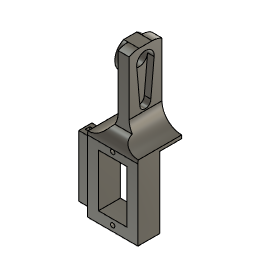
Final Assembly (Autodesk Fusion 360 archive; units mm, degrees)
design "hip_right_v2"
Autodesk Fusion 360 part; units mm, degrees
(part 1 of 2)
sketch "Sketch1" plane through (0, 0, 0) normal (1, 0, 0) x (0, 1, 0)
  line L0 (0, 0) -> (25, 0)
  line L1 (25, 0) -> (25, 35)
  line L2 (25, 35) -> (0, 35)
  line L3 (0, 35) -> (0, 0)
  dimension "d1" = 25
  dimension "d2" = 35
  constraint horizontal L0
  constraint vertical L1
  constraint horizontal L2
  constraint vertical L3
  constraint coincident L0.start L3.end
  measures "d1" distance of L0.start L0.end
  measures "d2" distance of L0.start L2.end
extrude "Extrude1" add sketch "Sketch1" along normal blind 5
sketch "Sketch2" plane through (5, 0, 0) normal (1, 0, 0) x (0, 1, 0)
  line L0 (0, 35) -> (0, 0)
  line L1 (0, 0) -> (25, 0)
  line L2 (25, 0) -> (25, 35)
  line L3 (25, 35) -> (0, 35)
  circle A0 centre (12.4718, 28.6693) radius 4
  line L4 (12.4317, 32.6691) -> (12.4317, 9.6691)
  circle A1 centre (12.4317, 12.1237) radius 2.5
  line L5 (14.9305, 12.1994) -> (16.454, 28.2923)
  line L6 (8.4897, 28.2923) -> (9.9414, 11.9031)
  line L7 (5, 35) -> (20, 35)
  line L8 (20, 35) -> (20, 0)
  line L9 (20, 0) -> (5, 0)
  line L10 (5, 0) -> (5, 35)
  dimension "d5" = 8
  dimension "d6" = 23
  dimension "d7" = 5
  constraint coincident A0 L4.start
  constraint vertical L4
  constraint coincident L4 A1.centre
  constraint coincident A1 L5.start
  constraint coincident A0 L5.end
  constraint tangent A0 L5
  constraint coincident A0 L6.start
  constraint coincident A1 L6.end
  constraint tangent A1 L6
  constraint horizontal L7
  constraint vertical L8
  constraint horizontal L9
  constraint vertical L10
  measures "d5" diameter of A0
  measures "d6" distance of L4.start L4.end
  measures "d7" diameter of A1
extrude "Extrude3" cut sketch "Sketch2" against normal blind 3 contours A0 L4 A1 L5 | A0 L4 A1 L6 | A1
extrude "Extrude2" cut sketch "Sketch2" against normal blind 5 contours A0 L4 | A0 L4
sketch "Sketch3" plane through (0, 0, 0) normal (-1, 0, 0) x (0, -1, 0)
  circle A0 centre (-12.4718, 28.6693) radius 4
  line L0 (0, 0) -> (0, 35)
  line L1 (0, 35) -> (-25, 35)
  line L2 (-25, 35) -> (-25, 0)
  line L3 (-25, 0) -> (0, 0)
  circle A1 centre (-12.4718, 28.6693) radius 4
  circle A2 centre (-12.4718, 28.6693) radius 7
  dimension "d12" = 14
  constraint concentric A0 A1
  constraint concentric A1 A2
  measures "d12" diameter of A2
extrude "Extrude4" add sketch "Sketch3" along normal blind 2 contours L1 A2 picked at (-12.3722, 34.2194)
sketch "Sketch4" plane through (0, 0, 0) normal (0, 0, -1) x (1, 0, 0)
  line L0 (0, 0) -> (0, -25)
  line L1 (0, -25) -> (5, -25)
  line L2 (5, -25) -> (5, 0)
  line L3 (5, 0) -> (0, 0)
  line L4 (0, 0) -> (5, 0)
  line L5 (5, 0) -> (5, -25)
  line L6 (5, -25) -> (0, -25)
  line L7 (0, -25) -> (0, 0)
  constraint horizontal L4
  constraint vertical L5
  constraint horizontal L6
  constraint vertical L7
  constraint coincident L1.end L2.start
  constraint coincident L0.start L3.end
extrude "Extrude5" add sketch "Sketch4" along normal blind 34
sketch "Sketch5" plane through (5, 0, 0) normal (1, 0, 0) x (0, 1, 0)
  arc A0 (16.454, 28.2923) -> (8.4897, 28.2923) centre (12.4718, 28.6693) ccw
  line L0 (16.454, 28.2923) -> (14.9305, 12.1994)
  arc A1 (9.9414, 11.9031) -> (14.9305, 12.1994) centre (12.4317, 12.1237) ccw
  line L1 (9.9414, 11.9031) -> (8.4897, 28.2923)
  line L2 (0, 35) -> (0, -34)
  line L3 (0, -34) -> (25, -34)
  line L4 (25, -34) -> (25, 35)
  line L5 (25, 35) -> (0, 35)
  line L6 (25, -34) -> (0, -34)
  line L7 (0, -34) -> (0, 0)
  line L8 (0, 0) -> (25, 0)
  line L9 (25, 0) -> (25, -34)
  constraint horizontal L6
  constraint vertical L7
  constraint horizontal L8
  constraint vertical L9
  constraint coincident L7.end L8.start
  constraint coincident L3.end L4.start
extrude "Extrude6" add sketch "Sketch5" along normal blind 12 contours L2 L3 L4 L6 L7 L8 L9
sketch "Sketch6" plane through (0, 0, 0) normal (-1, 0, 0) x (0, -1, 0)
  arc A0 (-15.4588, 35) -> (-9.4848, 35) centre (-12.4718, 28.6693) ccw
  line L0 (-15.4588, 35) -> (-25, 35)
  line L1 (-25, 35) -> (-25, -34)
  line L2 (-25, -34) -> (0, -34)
  line L3 (0, -34) -> (0, 35)
  line L4 (0, 35) -> (-9.4848, 35)
  line L5 (-25, -34) -> (0, -34)
  line L6 (0, -34) -> (0, 0)
  line L7 (0, 0) -> (-25, 0)
  line L8 (-25, 0) -> (-25, -34)
  constraint horizontal L5
  constraint vertical L6
  constraint horizontal L7
  constraint vertical L8
  constraint coincident L6.end L7.start
  constraint coincident L1.end L2.start
extrude "Extrude7" add sketch "Sketch6" along normal blind 12 contours L1 L2 L3 L5 L6 L7 L8
sketch "Sketch7" plane through (0, 25, 0) normal (0, 1, 0) x (-1, 0, 0)
  line L0 (0, 0) -> (0, 35)
  line L1 (0, 35) -> (-5, 35)
  line L2 (-5, 35) -> (-5, 0)
  line L3 (-5, 0) -> (-17, 0)
  line L4 (-17, 0) -> (-17, -34)
  line L5 (-17, -34) -> (12, -34)
  line L6 (12, -34) -> (12, 0)
  line L7 (12, 0) -> (0, 0)
  line L8 (-2.5, 0) -> (-2.5, -34)
  line L9 (-2.5, -34) -> (-2.5, -29)
  line L10 (-2.5, -29) -> (4, -29)
  line L11 (4, -29) -> (-9, -29)
  line L12 (-9, -29) -> (-9, -5)
  line L13 (-9, -5) -> (4, -5)
  line L14 (4, -5) -> (4, -29)
  dimension "d21" = 5
  dimension "d22" = 6.5
  dimension "d23" = 13
  dimension "d24" = 24
  constraint midpoint L5 L8.end
  constraint perpendicular L5 L9
  constraint perpendicular L9 L10
  constraint horizontal L11
  constraint vertical L12
  constraint horizontal L13
  constraint vertical L14
  measures "d21" distance of L8.end L9.end
  measures "d22" distance of L9.end L10.end
  measures "d23" distance of L10.end L11.end
  measures "d24" distance of L10.end L13.end
extrude "Extrude8" cut sketch "Sketch7" against normal blind 25 contours L8 L10 L11 L13 L14 | L8 L11 L12 L13
sketch "Sketch8" plane through (0, 25, 0) normal (0, 1, 0) x (-1, 0, 0)
  line L0 (-9, -29) -> (-9, -5)
  line L1 (-9, -5) -> (4, -5)
  line L2 (4, -5) -> (4, -29)
  line L3 (4, -29) -> (-9, -29)
  line L4 (0, 0) -> (0, 35)
  line L5 (0, 35) -> (-5, 35)
  line L6 (-5, 35) -> (-5, 0)
  line L7 (-5, 0) -> (-17, 0)
  line L8 (-17, 0) -> (-17, -34)
  line L9 (-17, -34) -> (12, -34)
  line L10 (12, -34) -> (12, 0)
  line L11 (12, 0) -> (0, 0)
  line L12 (-9, -5) -> (-14, -5)
  line L13 (-14, -5) -> (-14, 0)
  line L14 (-14, 0) -> (-9, 0)
  line L15 (-9, 0) -> (-9, -5)
  line L16 (4, -5) -> (9, -5)
  line L17 (9, -5) -> (9, 0)
  line L18 (9, 0) -> (4, 0)
  line L19 (4, 0) -> (4, -5)
  line L20 (9, 0) -> (12, 0)
  line L21 (12, 0) -> (12, -34)
  line L22 (12, -34) -> (9, -34)
  line L23 (9, -34) -> (9, 0)
  line L24 (-14, 0) -> (-17, 0)
  line L25 (-17, 0) -> (-17, -34)
  line L26 (-17, -34) -> (-14, -34)
  line L27 (-14, -34) -> (-14, 0)
  dimension "d27" = 5
  dimension "d28" = 5
  dimension "d29" = 5
  dimension "d30" = 5
  constraint horizontal L12
  constraint vertical L13
  constraint horizontal L14
  constraint vertical L15
  constraint coincident L0.end L1.start
  constraint horizontal L16
  constraint vertical L17
  constraint horizontal L18
  constraint vertical L19
  constraint coincident L1.end L2.start
  constraint horizontal L20
  constraint vertical L21
  constraint horizontal L22
  constraint vertical L23
  constraint coincident L9.end L10.start
  constraint horizontal L24
  constraint vertical L25
  constraint horizontal L26
  constraint vertical L27
  constraint coincident L8.end L9.start
  measures "d27" distance of L0.end L12.end
  measures "d28" distance of L0.end L14.end
  measures "d29" distance of L1.end L16.end
  measures "d30" distance of L1.end L18.end
extrude "Extrude9" cut sketch "Sketch8" against normal blind 25 contours L7 L8 L9 L13 L24 L25 L26 L27 | L9 L10 L11 L17 L20 L21 L22 L23
fillet "Fillet1" radius 9 2 edges at (5, 12.5, 0) (0, 12.5, 0)
sketch "Sketch9" plane through (0, 0, 0) normal (0, -1, 0) x (1, 0, 0)
  line L0 (9, -5) -> (9, -29)
  line L1 (9, -29) -> (-4, -29)
  line L2 (-4, -29) -> (-4, -5)
  line L3 (-4, -5) -> (9, -5)
  line L4 (-9, 0) -> (-9, -34)
  line L5 (-9, -34) -> (14, -34)
  line L6 (14, -34) -> (14, 0)
  arc A0 (5, 9) -> (14, 0) centre (14, 9) ccw
  line L7 (5, 9) -> (5, 35)
  line L8 (5, 35) -> (0, 35)
  line L9 (0, 35) -> (0, 9)
  arc A1 (-9, 0) -> (0, 9) centre (-9, 9) ccw
  line L10 (2.5, -29) -> (2.5, -31.5)
  line L11 (2.5, -5) -> (2.5, -2.5)
  circle A2 centre (2.5, -2.5) radius 1
  circle A3 centre (2.5, -31.5) radius 1
  dimension "d35" = 2.5
  dimension "d36" = 2.5
  dimension "d37" = 2
  dimension "d38" = 2
  constraint midpoint L1 L10.start
  constraint perpendicular L1 L10
  constraint midpoint L3 L11.start
  constraint perpendicular L3 L11
  constraint coincident L11.end A2.centre
  constraint coincident L10.end A3.centre
  measures "d35" distance of L10.start L10.end
  measures "d36" distance of L11.start L11.end
  measures "d37" diameter of A2
  measures "d38" diameter of A3
extrude "Extrude10" cut sketch "Sketch9" against normal blind 25 contours A2 | A3
sketch "Sketch10" plane through (0, 25, 0) normal (0, 1, 0) x (-1, 0, 0)
  circle A0 centre (-2.5, -31.5) radius 1
  circle A1 centre (-2.5, -2.5) radius 1
  line L0 (9, -34) -> (9, 0)
  arc A2 (0, 9) -> (9, 0) centre (9, 9) ccw
  line L1 (0, 9) -> (0, 35)
  line L2 (0, 35) -> (-5, 35)
  line L3 (-5, 35) -> (-5, 9)
  arc A3 (-14, 0) -> (-5, 9) centre (-14, 9) ccw
  line L4 (-14, 0) -> (-14, -34)
  line L5 (-14, -34) -> (9, -34)
  line L6 (-9, -29) -> (-9, -5)
  line L7 (-9, -5) -> (4, -5)
  line L8 (4, -5) -> (4, -29)
  line L9 (4, -29) -> (-9, -29)
  line L10 (-14, -34) -> (9, -34)
  line L11 (9, -34) -> (9, -1.4723)
  line L12 (9, -1.4723) -> (-14, -1.4723)
  line L13 (-14, -1.4723) -> (-14, -34)
  constraint horizontal L10
  constraint vertical L11
  constraint horizontal L12
  constraint vertical L13
  constraint coincident L0 L11.end
  constraint coincident L4.end L5.start
extrude "Extrude11" cut sketch "Sketch10" against normal blind 15 contours L0 L4 L5 L10 L11 L12 L13
fillet "Fillet2" radius 9.5 2 edges at (2.5, 0, 35) (2.5, 25, 35)
sketch "Sketch11" plane through (14, 0, 0) normal (1, 0, 0) x (0, 1, 0)
  line L0 (10, -34) -> (10, -1.4723)
  line L1 (10, -1.4723) -> (25, -1.4723)
  line L2 (25, -1.4723) -> (25, 0)
  line L3 (25, 0) -> (0, 0)
  line L4 (0, 0) -> (0, -34)
  line L5 (0, -34) -> (10, -34)
  line L6 (0, 5) -> (5, 5)
  line L7 (5, 5) -> (5, 35)
  line L8 (5, 35) -> (0, 35)
  line L9 (0, 35) -> (0, 5)
  line L10 (25, 5) -> (20, 5)
  line L11 (20, 5) -> (20, 35)
  line L12 (20, 35) -> (25, 35)
  line L13 (25, 35) -> (25, 5)
  constraint horizontal L6
  constraint vertical L7
  constraint horizontal L8
  constraint vertical L9
  constraint horizontal L10
  constraint vertical L11
  constraint horizontal L12
  constraint vertical L13
extrude "Extrude12" cut sketch "Sketch11" against normal blind 19 contours L6 L7 L8 L9 | L10 L11 L12 L13
sketch "Sketch12" plane through (14, 0, 0) normal (1, 0, 0) x (0, 1, 0)
  line L0 (10, -34) -> (10, -1.4723)
  line L1 (10, -1.4723) -> (25, -1.4723)
  line L2 (25, -1.4723) -> (25, 0)
  line L3 (25, 0) -> (0, 0)
  line L4 (0, 0) -> (0, -34)
  line L5 (0, -34) -> (10, -34)
  line L6 (20, 5) -> (25, 5)
  line L7 (25, 5) -> (25, -1.4723)
  line L8 (25, -1.4723) -> (20, -1.4723)
  line L9 (20, -1.4723) -> (20, 5)
  constraint horizontal L6
  constraint vertical L7
  constraint horizontal L8
  constraint vertical L9
  constraint coincident L1.end L2.start
extrude "Extrude13" cut sketch "Sketch12" against normal blind 23 contours L1 L2 L3 L7 L8 L9 | L3 L6 L7 L9
sketch "Sketch14" plane through (14, 0, 0) normal (1, 0, 0) x (0, 1, 0)
  line L0 (0, 0) -> (0, -34)
  line L1 (0, -34) -> (10, -34)
  line L2 (10, -34) -> (10, -1.4723)
  line L3 (10, -1.4723) -> (20, -1.4723)
  line L4 (20, -1.4723) -> (20, 0)
  line L5 (20, 0) -> (0, 0)
  line L6 (5, 9) -> (0, 9)
  line L7 (0, 9) -> (0, 4)
  line L8 (0, 4) -> (5, 4)
  line L9 (5, 4) -> (5, 9)
  dimension "d55" = 5
  constraint horizontal L6
  constraint vertical L7
  constraint horizontal L8
  constraint vertical L9
  measures "d55" distance of L6.start L6.end
extrude "Extrude15" cut sketch "Sketch14" against normal blind 18 contours L6 L7 L8 L9
fillet "Fillet5" radius 5.5 1 edges at (2.5, 0, 4)
sketch "Sketch15" plane through (-9, 0, 0) normal (-1, 0, 0) x (0, -1, 0)
  arc A0 (0, -1.4772) -> (-0.2021, 0) centre (-5.5, -1.4772) ccw
  line L0 (-0.2021, 0) -> (-20, 0)
  line L1 (-20, 0) -> (-20, -1.4723)
  line L2 (-20, -1.4723) -> (-10, -1.4723)
  line L3 (-10, -1.4723) -> (-10, -34)
  line L4 (-10, -34) -> (0, -34)
  line L5 (0, -34) -> (0, -1.4772)
  line L6 (0, -17.7386) -> (-2, -17.7386)
  line L7 (-2, -17.7386) -> (-8, -17.7386)
  line L8 (-8, -17.7386) -> (-8, -3.7386)
  line L9 (-8, -3.7386) -> (-2, -3.7386)
  line L10 (-2, -3.7386) -> (-2, -17.7386)
  line L11 (-2, -17.7386) -> (-8, -17.7386)
  line L12 (-8, -17.7386) -> (-8, -31.7386)
  line L13 (-8, -31.7386) -> (-2, -31.7386)
  line L14 (-2, -31.7386) -> (-2, -17.7386)
  dimension "d64" = 2
  dimension "d65" = 6
  dimension "d66" = 14
  dimension "d67" = 14
  constraint midpoint L5 L6.start
  constraint perpendicular L5 L6
  constraint horizontal L7
  constraint vertical L8
  constraint horizontal L9
  constraint vertical L10
  constraint horizontal L11
  constraint vertical L12
  constraint horizontal L13
  constraint vertical L14
  measures "d64" distance of L6.start L6.end
  measures "d65" distance of L6.end L7.end
  measures "d66" distance of L6.end L9.end
  measures "d67" distance of L6.end L13.end
extrude "Extrude16" add sketch "Sketch15" along normal blind 6 contours L7 L11 L12 L13 L14 | L7 L8 L9 L10 L11
sketch "Sketch16" plane through (0, 0, -3.7386) normal (0, 0, 1) x (-1, 0, 0)
  line L0 (9, -2) -> (9, -8)
  line L1 (9, -8) -> (15, -8)
  line L2 (15, -8) -> (15, -2)
  line L3 (15, -2) -> (9, -2)
  line L4 (9, -8) -> (12, -8)
  line L5 (12, -8) -> (12, -4)
  line L6 (12, -4) -> (9, -4)
  line L7 (9, -4) -> (9, -8)
  line L8 (12, -4) -> (14, -4)
  line L9 (14, -4) -> (14, -6)
  line L10 (14, -6) -> (12, -6)
  line L11 (12, -6) -> (12, -4)
  dimension "d70" = 3
  dimension "d71" = 4
  dimension "d74" = 2
  dimension "d75" = 2
  constraint horizontal L4
  constraint vertical L5
  constraint horizontal L6
  constraint vertical L7
  constraint coincident L0.end L1.start
  constraint horizontal L8
  constraint vertical L9
  constraint horizontal L10
  constraint vertical L11
  measures "d70" distance of L0.end L4.end
  measures "d71" distance of L0.end L6.end
  measures "d74" distance of L5.end L8.end
  measures "d75" distance of L5.end L10.end
extrude "Extrude18" cut sketch "Sketch16" against normal blind 28 contours L0 L1 L4 L5 L6 L7 L11 | L5 L8 L9 L10 L11
extrude "Extrude17" cut sketch "Sketch16" against normal blind 28 contours L0 L1 L4 L5 L6 L7 L11

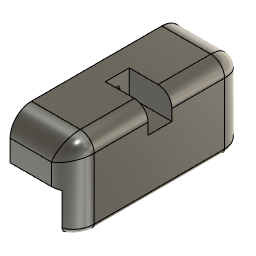
design "face_plate"
Autodesk Fusion 360 part; units mm, degrees
sketch "Sketch1" plane through (0, 0, 0) normal (1, 0, 0) x (0, 1, 0)
  line L0 (0, 0) -> (69, 0)
  line L1 (69, 0) -> (69, 32)
  line L2 (69, 32) -> (0, 32)
  line L3 (0, 32) -> (0, 0)
  dimension "d1" = 69
  dimension "d2" = 32
  constraint horizontal L0
  constraint vertical L1
  constraint horizontal L2
  constraint vertical L3
  constraint coincident L0.start L3.end
  measures "d1" distance of L0.start L0.end
  measures "d2" distance of L0.start L2.end
extrude "Extrude1" add sketch "Sketch1" along normal blind 20
sketch "Sketch3" plane through (0, 0, 0) normal (-1, 0, 0) x (0, -1, 0)
  line L0 (0, 0) -> (0, 32)
  line L1 (0, 32) -> (-69, 32)
  line L2 (-69, 32) -> (-69, 0)
  line L3 (-69, 0) -> (0, 0)
  line L4 (-69, 0) -> (-35, 0)
  line L5 (-35, 0) -> (-35, 9.9631)
  line L6 (-35, 9.9631) -> (-69, 9.9631)
  line L7 (-69, 9.9631) -> (-69, 0)
  constraint horizontal L4
  constraint vertical L5
  constraint horizontal L6
  constraint vertical L7
  constraint coincident L2.end L3.start
sketch "Sketch4" plane through (20, 0, 0) normal (1, 0, 0) x (0, 1, 0)
  line L0 (0, 32) -> (0, 0)
  line L1 (0, 0) -> (69, 0)
  line L2 (69, 0) -> (69, 32)
  line L3 (69, 32) -> (0, 32)
  line L4 (34.5, 32) -> (39.5, 32)
  line L5 (39.5, 32) -> (39.5, 26)
  line L6 (39.5, 26) -> (34.5, 26)
  line L7 (34.5, 26) -> (34.5, 32)
  line L8 (39.5, 26) -> (34.5, 26)
  line L9 (34.5, 26) -> (34.5, 22)
  line L10 (34.5, 22) -> (39.5, 22)
  line L11 (39.5, 22) -> (39.5, 26)
  line L12 (34.5, 32) -> (30, 32)
  line L13 (30, 32) -> (30, 22)
  line L14 (30, 22) -> (34.5, 22)
  line L15 (34.5, 22) -> (34.5, 32)
  dimension "d18" = 5
  dimension "d19" = 6
  dimension "d20" = 4
  constraint horizontal L4
  constraint vertical L5
  constraint horizontal L6
  constraint vertical L7
  constraint midpoint L3 L4.start
  constraint horizontal L8
  constraint vertical L9
  constraint horizontal L10
  constraint vertical L11
  constraint horizontal L12
  constraint vertical L13
  constraint horizontal L14
  constraint vertical L15
  measures "d18" distance of L4.start L4.end
  measures "d19" distance of L4.start L6.end
  measures "d20" distance of L5.end L10.end
extrude "Extrude4" cut sketch "Sketch4" against normal blind 17 contours L3 L7 L9 L12 L13 L14 L15 | L3 L4 L5 L6 L7 L8 L15 | L6 L8 L9 L10 L11 L15
sketch "Sketch5" plane through (3, 0, 0) normal (1, 0, 0) x (0, 1, 0)
  line L0 (39.5, 32) -> (30, 32)
  line L1 (30, 32) -> (30, 22)
  line L2 (30, 22) -> (39.5, 22)
  line L3 (39.5, 22) -> (39.5, 32)
  line L4 (34.75, 32) -> (34.75, 27)
  circle A0 centre (34.75, 27) radius 1
  dimension "d23" = 5
  dimension "d24" = 2
  constraint midpoint L0 L4.start
  constraint perpendicular L0 L4
  constraint coincident L4.end A0.centre
  measures "d23" distance of L4.start L4.end
  measures "d24" diameter of A0
extrude "Extrude5" cut sketch "Sketch5" against normal blind 3 contours A0
fillet "Fillet1" radius 5.5 2 edges at (20, 15, 32) (20, 54.25, 32)
fillet "Fillet2" radius 8.5 6 edges at (7.25, 0, 32) (18.3891, 0, 30.3891) (20, 0, 13.25) (20, 69, 13.25) (18.3891, 69, 30.3891) (7.25, 69, 32)
sketch "Sketch7" plane through (0, 0, 0) normal (-1, 0, 0) x (0, -1, 0)
  arc A0 (-60.5, 32) -> (-69, 23.5) centre (-60.5, 23.5) ccw
  line L0 (-69, 23.5) -> (-69, 0)
  line L1 (-69, 0) -> (0, 0)
  line L2 (0, 0) -> (0, 23.5)
  arc A1 (0, 23.5) -> (-8.5, 32) centre (-8.5, 23.5) ccw
  line L3 (-8.5, 32) -> (-60.5, 32)
  circle A2 centre (-34.75, 27) radius 1
  line L4 (-69, 0) -> (-65, 0)
  line L5 (-65, 0) -> (-65, 15)
  line L6 (-65, 15) -> (-69, 15)
  line L7 (-69, 15) -> (-69, 0)
  line L8 (0, 0) -> (-4, 0)
  line L9 (-4, 0) -> (-4, 15)
  line L10 (-4, 15) -> (0, 15)
  line L11 (0, 15) -> (0, 0)
  line L12 (-65, 0) -> (-42.5, 0)
  line L13 (-42.5, 0) -> (-42.5, 25)
  line L14 (-42.5, 25) -> (-65, 25)
  line L15 (-65, 25) -> (-65, 0)
  line L16 (-4, 0) -> (-26.5, 0)
  line L17 (-26.5, 0) -> (-26.5, 25)
  line L18 (-26.5, 25) -> (-4, 25)
  line L19 (-4, 25) -> (-4, 0)
  dimension "d39" = 4
  dimension "d40" = 4
  dimension "d41" = 15
  dimension "d42" = 25
  dimension "d43" = 22.5
  dimension "d44" = 22.5
  dimension "d45" = 25
  constraint horizontal L4
  constraint vertical L5
  constraint horizontal L6
  constraint vertical L7
  constraint coincident L0.end L1.start
  constraint horizontal L8
  constraint vertical L9
  constraint horizontal L10
  constraint vertical L11
  constraint coincident L1.end L2.start
  constraint horizontal L12
  constraint vertical L13
  constraint horizontal L14
  constraint vertical L15
  constraint horizontal L16
  constraint vertical L17
  constraint horizontal L18
  constraint vertical L19
  measures "d39" distance of L0.end L4.end
  measures "d40" distance of L1.end L8.end
  measures "d41" distance of L1.end L10.end
  measures "d42" distance of L12.end L13.end
  measures "d43" distance of L13.end L14.end
  measures "d44" distance of L8.end L16.end
  measures "d45" distance of L8.end L18.end
extrude "Extrude7" cut sketch "Sketch7" against normal blind 9.5 contours L0 L1 L4 L5 L6 L7 L15 | L1 L5 L12 L13 L14 L15 | L1 L2 L8 L9 L10 L11 L19 | L1 L9 L16 L17 L18 L19
sketch "Sketch8" plane through (0, 0, 0) normal (-1, 0, 0) x (0, -1, 0)
  line L0 (-42.5, 25) -> (-42.5, 0)
  line L1 (-42.5, 0) -> (-26.5, 0)
  line L2 (-26.5, 0) -> (-26.5, 25)
  line L3 (-26.5, 25) -> (-4, 25)
  line L4 (-4, 25) -> (-4, 15)
  line L5 (-4, 15) -> (0, 15)
  line L6 (0, 15) -> (0, 23.5)
  arc A0 (0, 23.5) -> (-8.5, 32) centre (-8.5, 23.5) ccw
  line L7 (-8.5, 32) -> (-60.5, 32)
  arc A1 (-60.5, 32) -> (-69, 23.5) centre (-60.5, 23.5) ccw
  line L8 (-69, 23.5) -> (-69, 15)
  line L9 (-69, 15) -> (-65, 15)
  line L10 (-65, 15) -> (-65, 25)
  line L11 (-65, 25) -> (-42.5, 25)
  circle A2 centre (-34.75, 27) radius 1
  line L12 (-26.5, 25) -> (-26.5, 0)
  line L13 (-26.5, 0) -> (-42.5, 0)
  line L14 (-42.5, 0) -> (-42.5, 25)
  line L15 (-26.5, 20.102) -> (-42.5, 20.102)
  constraint vertical L12
  constraint horizontal L13
  constraint vertical L14
  constraint coincident L1.end L2.start
  constraint coincident L0.start L11.end
  constraint coincident L12 L15.start
  constraint coincident L14 L15.end
  constraint perpendicular L14 L15
extrude "Extrude8" cut sketch "Sketch8" against normal blind 15.5 contours L0 L1 L2 L12 L13 L14 L15
sketch "Sketch9" plane through (9.5, 0, 0) normal (-1, 0, 0) x (0, -1, 0)
  line L0 (-65, 25) -> (-65, 15)
  line L1 (-65, 15) -> (-69, 15)
  line L2 (-69, 15) -> (-69, 0)
  line L3 (-69, 0) -> (-42.5, 0)
  line L4 (-42.5, 0) -> (-42.5, 20.102)
  line L5 (-42.5, 20.102) -> (-42.5, 25)
  line L6 (-42.5, 25) -> (-65, 25)
  line L7 (-42.5, 0) -> (-62.5, 0)
  line L8 (-62.5, 0) -> (-62.5, 20)
  line L9 (-62.5, 20) -> (-42.5, 20)
  line L10 (-42.5, 20) -> (-42.5, 0)
  line L11 (-26.5, 0) -> (-6.5, 0)
  line L12 (-6.5, 0) -> (-6.5, 20)
  line L13 (-6.5, 20) -> (-26.5, 20)
  line L14 (-26.5, 20) -> (-26.5, 0)
  dimension "d50" = 20
  dimension "d51" = 20
  constraint horizontal L7
  constraint vertical L8
  constraint horizontal L9
  constraint vertical L10
  constraint coincident L3.end L4.start
  constraint horizontal L11
  constraint vertical L12
  constraint horizontal L13
  constraint vertical L14
  measures "d50" distance of L8.end L9.end
  measures "d51" distance of L7.end L8.end
extrude "Extrude9" cut sketch "Sketch9" against normal blind 7.5 contours L3 L4 L7 L8 L9 L10 | L11 L12 L13 L14
fillet "Fillet4" radius 2 5 edges at (10.5, 0, 0) (17.5104, 2.4896, 0) (20, 34.5, 0) (17.5104, 66.5104, 0) (10.5, 69, 0)
sketch "Sketch10" plane through (0, 0, 0) normal (-1, 0, 0) x (0, -1, 0)
  circle A0 centre (-34.75, 27) radius 1
  line L0 (-42.5, 20.102) -> (-26.5, 20.102)
  line L1 (-26.5, 20.102) -> (-26.5, 25)
  line L2 (-26.5, 25) -> (-4, 25)
  line L3 (-4, 25) -> (-4, 15)
  line L4 (-4, 15) -> (0, 15)
  line L5 (0, 15) -> (0, 23.5)
  arc A1 (0, 23.5) -> (-8.5, 32) centre (-8.5, 23.5) ccw
  line L6 (-8.5, 32) -> (-60.5, 32)
  arc A2 (-60.5, 32) -> (-69, 23.5) centre (-60.5, 23.5) ccw
  line L7 (-69, 23.5) -> (-69, 15)
  line L8 (-69, 15) -> (-65, 15)
  line L9 (-65, 15) -> (-65, 25)
  line L10 (-65, 25) -> (-42.5, 25)
  line L11 (-42.5, 25) -> (-42.5, 20.102)
  line L12 (-70, 32.5) -> (2, 32.5)
  line L13 (2, 32.5) -> (2, 15)
  line L14 (2, 15) -> (-70, 15)
  line L15 (-70, 15) -> (-70, 32.5)
  constraint horizontal L12
  constraint vertical L13
  constraint horizontal L14
  constraint vertical L15
extrude "Extrude10" add sketch "Sketch10" along normal blind 5 contours L0 L1 L2 L3 L4 L5 A1 L6 A2 L7 L8 L9 L10 L11 L14
sketch "Sketch11" plane through (0, 0, 0) normal (0, -1, 0) x (1, 0, 0)
  line L0 (9.5, 2) -> (11.5, 2)
  line L1 (11.5, 2) -> (11.5, 23.5)
  line L2 (11.5, 23.5) -> (-5, 23.5)
  line L3 (-5, 23.5) -> (-5, 15)
  line L4 (-5, 15) -> (9.5, 15)
  line L5 (9.5, 15) -> (9.5, 2)
  line L6 (9.5, 0) -> (15, 0)
  line L7 (15, 0) -> (15, 15)
  line L8 (15, 15) -> (9.5, 15)
  line L9 (9.5, 15) -> (9.5, 0)
  constraint horizontal L6
  constraint vertical L7
  constraint horizontal L8
  constraint vertical L9
extrude "Extrude11" cut sketch "Sketch11" against normal blind 69.5 contours L0 L1 L5 L8 L9 | L0 L1 L6 L7 L8 L9

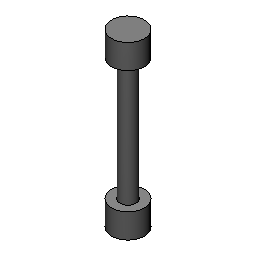
design "pin"
Autodesk Fusion 360 part; units mm, degrees
sketch "Sketch1" plane through (0, 0, 0) normal (0, 0, 1) x (1, 0, 0)
  circle A0 centre (0, 0) radius 2
  dimension "d1" = 4
  constraint coincident A0.centre origin
  measures "d1" diameter of A0
extrude "Extrude1" add sketch "Sketch1" along normal blind 3
sketch "Sketch2" plane through (0, 0, 0) normal (0, 1, 0) x (1, 0, 0)
sketch "Sketch3" plane through (0, 0, 3) normal (0, 0, 1) x (-1, 0, 0)
  circle A0 centre (0, 0) radius 2
  circle A1 centre (0, 0) radius 1
  dimension "d4" = 2
  constraint coincident A0.centre A1.centre
  measures "d4" diameter of A1
extrude "Extrude2" add sketch "Sketch3" along normal blind 15 contours A1
sketch "Sketch4" plane through (0, 0, 18) normal (0, 0, 1) x (-1, 0, 0)
  circle A0 centre (0, 0) radius 1
  circle A1 centre (0, 0) radius 2
  dimension "d7" = 4
  constraint concentric A0 A1
  measures "d7" diameter of A1
extrude "Extrude3" add sketch "Sketch4" along normal blind 3 contours A0 | A1

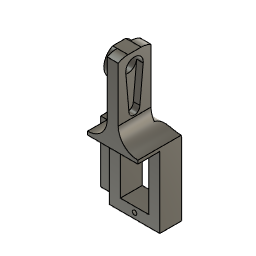
design "hip_left_v2"
Autodesk Fusion 360 part; units mm, degrees
sketch "Sketch1" plane through (0, 0, 0) normal (1, 0, 0) x (0, 1, 0)
  line L0 (0, 0) -> (25, 0)
  line L1 (25, 0) -> (25, 35)
  line L2 (25, 35) -> (0, 35)
  line L3 (0, 35) -> (0, 0)
  dimension "d1" = 25
  dimension "d2" = 35
  constraint horizontal L0
  constraint vertical L1
  constraint horizontal L2
  constraint vertical L3
  constraint coincident L0.start L3.end
  measures "d1" distance of L0.start L0.end
  measures "d2" distance of L0.start L2.end
extrude "Extrude1" add sketch "Sketch1" along normal blind 5
sketch "Sketch2" plane through (5, 0, 0) normal (1, 0, 0) x (0, 1, 0)
  line L0 (0, 35) -> (0, 0)
  line L1 (0, 0) -> (25, 0)
  line L2 (25, 0) -> (25, 35)
  line L3 (25, 35) -> (0, 35)
  circle A0 centre (12.4718, 28.6693) radius 4
  line L4 (12.4317, 32.6691) -> (12.4317, 9.6691)
  circle A1 centre (12.4317, 12.1237) radius 2.5
  line L5 (14.9305, 12.1994) -> (16.454, 28.2923)
  line L6 (8.4897, 28.2923) -> (9.9414, 11.9031)
  dimension "d5" = 8
  dimension "d6" = 23
  dimension "d7" = 5
  constraint coincident A0 L4.start
  constraint vertical L4
  constraint coincident L4 A1.centre
  constraint coincident A1 L5.start
  constraint coincident A0 L5.end
  constraint tangent A0 L5
  constraint coincident A0 L6.start
  constraint coincident A1 L6.end
  constraint tangent A1 L6
  measures "d5" diameter of A0
  measures "d6" distance of L4.start L4.end
  measures "d7" diameter of A1
extrude "Extrude3" cut sketch "Sketch2" against normal blind 3 contours A0 L4 A1 L5 | A0 L4 A1 L6 | A1
extrude "Extrude2" cut sketch "Sketch2" against normal blind 5 contours A0 L4 | A0 L4
sketch "Sketch3" plane through (0, 0, 0) normal (-1, 0, 0) x (0, -1, 0)
  circle A0 centre (-12.4718, 28.6693) radius 4
  line L0 (0, 0) -> (0, 35)
  line L1 (0, 35) -> (-25, 35)
  line L2 (-25, 35) -> (-25, 0)
  line L3 (-25, 0) -> (0, 0)
  circle A1 centre (-12.4718, 28.6693) radius 4
  circle A2 centre (-12.4718, 28.6693) radius 7
  dimension "d12" = 14
  constraint concentric A0 A1
  constraint concentric A1 A2
  measures "d12" diameter of A2
extrude "Extrude4" add sketch "Sketch3" along normal blind 2 contours L1 A2 picked at (-12.3722, 34.2194)
sketch "Sketch4" plane through (0, 0, 0) normal (0, 0, -1) x (1, 0, 0)
  line L0 (0, 0) -> (0, -25)
  line L1 (0, -25) -> (5, -25)
  line L2 (5, -25) -> (5, 0)
  line L3 (5, 0) -> (0, 0)
  line L4 (0, 0) -> (5, 0)
  line L5 (5, 0) -> (5, -25)
  line L6 (5, -25) -> (0, -25)
  line L7 (0, -25) -> (0, 0)
  constraint horizontal L4
  constraint vertical L5
  constraint horizontal L6
  constraint vertical L7
  constraint coincident L1.end L2.start
  constraint coincident L0.start L3.end
extrude "Extrude5" add sketch "Sketch4" along normal blind 34
sketch "Sketch5" plane through (5, 0, 0) normal (1, 0, 0) x (0, 1, 0)
  arc A0 (16.454, 28.2923) -> (8.4897, 28.2923) centre (12.4718, 28.6693) ccw
  line L0 (16.454, 28.2923) -> (14.9305, 12.1994)
  arc A1 (9.9414, 11.9031) -> (14.9305, 12.1994) centre (12.4317, 12.1237) ccw
  line L1 (9.9414, 11.9031) -> (8.4897, 28.2923)
  line L2 (0, 35) -> (0, -34)
  line L3 (0, -34) -> (25, -34)
  line L4 (25, -34) -> (25, 35)
  line L5 (25, 35) -> (0, 35)
  line L6 (25, -34) -> (0, -34)
  line L7 (0, -34) -> (0, 0)
  line L8 (0, 0) -> (25, 0)
  line L9 (25, 0) -> (25, -34)
  constraint horizontal L6
  constraint vertical L7
  constraint horizontal L8
  constraint vertical L9
  constraint coincident L7.end L8.start
  constraint coincident L3.end L4.start
extrude "Extrude6" add sketch "Sketch5" along normal blind 12 contours L2 L3 L4 L6 L7 L8 L9
sketch "Sketch6" plane through (0, 0, 0) normal (-1, 0, 0) x (0, -1, 0)
  arc A0 (-15.4588, 35) -> (-9.4848, 35) centre (-12.4718, 28.6693) ccw
  line L0 (-15.4588, 35) -> (-25, 35)
  line L1 (-25, 35) -> (-25, -34)
  line L2 (-25, -34) -> (0, -34)
  line L3 (0, -34) -> (0, 35)
  line L4 (0, 35) -> (-9.4848, 35)
  line L5 (-25, -34) -> (0, -34)
  line L6 (0, -34) -> (0, 0)
  line L7 (0, 0) -> (-25, 0)
  line L8 (-25, 0) -> (-25, -34)
  constraint horizontal L5
  constraint vertical L6
  constraint horizontal L7
  constraint vertical L8
  constraint coincident L6.end L7.start
  constraint coincident L1.end L2.start
extrude "Extrude7" add sketch "Sketch6" along normal blind 12 contours L1 L2 L3 L5 L6 L7 L8
sketch "Sketch7" plane through (0, 25, 0) normal (0, 1, 0) x (-1, 0, 0)
  line L0 (0, 0) -> (0, 35)
  line L1 (0, 35) -> (-5, 35)
  line L2 (-5, 35) -> (-5, 0)
  line L3 (-5, 0) -> (-17, 0)
  line L4 (-17, 0) -> (-17, -34)
  line L5 (-17, -34) -> (12, -34)
  line L6 (12, -34) -> (12, 0)
  line L7 (12, 0) -> (0, 0)
  line L8 (-2.5, 0) -> (-2.5, -34)
  line L9 (-2.5, -34) -> (-2.5, -29)
  line L10 (-2.5, -29) -> (4, -29)
  line L11 (4, -29) -> (-9, -29)
  line L12 (-9, -29) -> (-9, -5)
  line L13 (-9, -5) -> (4, -5)
  line L14 (4, -5) -> (4, -29)
  dimension "d21" = 5
  dimension "d22" = 6.5
  dimension "d23" = 13
  dimension "d24" = 24
  constraint midpoint L5 L8.end
  constraint perpendicular L5 L9
  constraint perpendicular L9 L10
  constraint horizontal L11
  constraint vertical L12
  constraint horizontal L13
  constraint vertical L14
  measures "d21" distance of L8.end L9.end
  measures "d22" distance of L9.end L10.end
  measures "d23" distance of L10.end L11.end
  measures "d24" distance of L10.end L13.end
extrude "Extrude8" cut sketch "Sketch7" against normal blind 25 contours L8 L10 L11 L13 L14 | L8 L11 L12 L13
sketch "Sketch8" plane through (0, 25, 0) normal (0, 1, 0) x (-1, 0, 0)
  line L0 (-9, -29) -> (-9, -5)
  line L1 (-9, -5) -> (4, -5)
  line L2 (4, -5) -> (4, -29)
  line L3 (4, -29) -> (-9, -29)
  line L4 (0, 0) -> (0, 35)
  line L5 (0, 35) -> (-5, 35)
  line L6 (-5, 35) -> (-5, 0)
  line L7 (-5, 0) -> (-17, 0)
  line L8 (-17, 0) -> (-17, -34)
  line L9 (-17, -34) -> (12, -34)
  line L10 (12, -34) -> (12, 0)
  line L11 (12, 0) -> (0, 0)
  line L12 (-9, -5) -> (-14, -5)
  line L13 (-14, -5) -> (-14, 0)
  line L14 (-14, 0) -> (-9, 0)
  line L15 (-9, 0) -> (-9, -5)
  line L16 (4, -5) -> (9, -5)
  line L17 (9, -5) -> (9, 0)
  line L18 (9, 0) -> (4, 0)
  line L19 (4, 0) -> (4, -5)
  line L20 (9, 0) -> (12, 0)
  line L21 (12, 0) -> (12, -34)
  line L22 (12, -34) -> (9, -34)
  line L23 (9, -34) -> (9, 0)
  line L24 (-14, 0) -> (-17, 0)
  line L25 (-17, 0) -> (-17, -34)
  line L26 (-17, -34) -> (-14, -34)
  line L27 (-14, -34) -> (-14, 0)
  dimension "d27" = 5
  dimension "d28" = 5
  dimension "d29" = 5
  dimension "d30" = 5
  constraint horizontal L12
  constraint vertical L13
  constraint horizontal L14
  constraint vertical L15
  constraint coincident L0.end L1.start
  constraint horizontal L16
  constraint vertical L17
  constraint horizontal L18
  constraint vertical L19
  constraint coincident L1.end L2.start
  constraint horizontal L20
  constraint vertical L21
  constraint horizontal L22
  constraint vertical L23
  constraint coincident L9.end L10.start
  constraint horizontal L24
  constraint vertical L25
  constraint horizontal L26
  constraint vertical L27
  constraint coincident L8.end L9.start
  measures "d27" distance of L0.end L12.end
  measures "d28" distance of L0.end L14.end
  measures "d29" distance of L1.end L16.end
  measures "d30" distance of L1.end L18.end
extrude "Extrude9" cut sketch "Sketch8" against normal blind 25 contours L7 L8 L9 L13 L24 L25 L26 L27 | L9 L10 L11 L17 L20 L21 L22 L23
fillet "Fillet1" radius 9 2 edges at (5, 12.5, 0) (0, 12.5, 0)
sketch "Sketch9" plane through (0, 0, 0) normal (0, -1, 0) x (1, 0, 0)
  line L0 (9, -5) -> (9, -29)
  line L1 (9, -29) -> (-4, -29)
  line L2 (-4, -29) -> (-4, -5)
  line L3 (-4, -5) -> (9, -5)
  line L4 (-9, 0) -> (-9, -34)
  line L5 (-9, -34) -> (14, -34)
  line L6 (14, -34) -> (14, 0)
  arc A0 (5, 9) -> (14, 0) centre (14, 9) ccw
  line L7 (5, 9) -> (5, 35)
  line L8 (5, 35) -> (0, 35)
  line L9 (0, 35) -> (0, 9)
  arc A1 (-9, 0) -> (0, 9) centre (-9, 9) ccw
  line L10 (2.5, -29) -> (2.5, -31.5)
  line L11 (2.5, -5) -> (2.5, -2.5)
  circle A2 centre (2.5, -2.5) radius 1
  circle A3 centre (2.5, -31.5) radius 1
  dimension "d35" = 2.5
  dimension "d36" = 2.5
  dimension "d37" = 2
  dimension "d38" = 2
  constraint midpoint L1 L10.start
  constraint perpendicular L1 L10
  constraint midpoint L3 L11.start
  constraint perpendicular L3 L11
  constraint coincident L11.end A2.centre
  constraint coincident L10.end A3.centre
  measures "d35" distance of L10.start L10.end
  measures "d36" distance of L11.start L11.end
  measures "d37" diameter of A2
  measures "d38" diameter of A3
extrude "Extrude10" cut sketch "Sketch9" against normal blind 25 contours A2 | A3
sketch "Sketch10" plane through (0, 0, 0) normal (0, -1, 0) x (1, 0, 0)
  circle A0 centre (2.5, -31.5) radius 1
  circle A1 centre (2.5, -2.5) radius 1
  line L0 (9, -5) -> (9, -29)
  line L1 (9, -29) -> (-4, -29)
  line L2 (-4, -29) -> (-4, -5)
  line L3 (-4, -5) -> (9, -5)
  line L4 (-9, 0) -> (-9, -34)
  line L5 (-9, -34) -> (14, -34)
  line L6 (14, -34) -> (14, 0)
  arc A2 (5, 9) -> (14, 0) centre (14, 9) ccw
  line L7 (5, 9) -> (5, 35)
  line L8 (5, 35) -> (0, 35)
  line L9 (0, 35) -> (0, 9)
  arc A3 (-9, 0) -> (0, 9) centre (-9, 9) ccw
  line L10 (14, -34) -> (-9, -34)
  line L11 (-9, -34) -> (-9, -1.5369)
  line L12 (-9, -1.5369) -> (14, -1.5369)
  line L13 (14, -1.5369) -> (14, -34)
  constraint horizontal L10
  constraint vertical L11
  constraint horizontal L12
  constraint vertical L13
  constraint coincident L4 L11.end
  constraint coincident L5.end L6.start
extrude "Extrude11" cut sketch "Sketch10" against normal blind 15 contours A1 L4 L5 L6 L10 L11 L12 L13
fillet "Fillet2" radius 9.5 2 edges at (2.5, 25, 35) (2.5, 0, 35)
sketch "Sketch11" plane through (14, 0, 0) normal (1, 0, 0) x (0, 1, 0)
  line L0 (0, -1.5369) -> (15, -1.5369)
  line L1 (15, -1.5369) -> (15, -34)
  line L2 (15, -34) -> (25, -34)
  line L3 (25, -34) -> (25, 0)
  line L4 (25, 0) -> (0, 0)
  line L5 (0, 0) -> (0, -1.5369)
  line L6 (25, 9) -> (20, 9)
  line L7 (20, 9) -> (20, 34)
  line L8 (20, 34) -> (25, 34)
  line L9 (25, 34) -> (25, 9)
  line L10 (0, 9) -> (5, 9)
  line L11 (5, 9) -> (5, 34)
  line L12 (5, 34) -> (0, 34)
  line L13 (0, 34) -> (0, 9)
  dimension "d45" = 5
  dimension "d46" = 25
  constraint horizontal L6
  constraint vertical L7
  constraint horizontal L8
  constraint vertical L9
  constraint horizontal L10
  constraint vertical L11
  constraint horizontal L12
  constraint vertical L13
  measures "d45" distance of L6.start L6.end
  measures "d46" distance of L6.start L8.end
extrude "Extrude12" cut sketch "Sketch11" against normal blind 20 contours L6 L7 L8 L9 | L10 L11 L12 L13
sketch "Sketch12" plane through (14, 0, 0) normal (1, 0, 0) x (0, 1, 0)
  line L0 (0, -1.5369) -> (15, -1.5369)
  line L1 (15, -1.5369) -> (15, -34)
  line L2 (15, -34) -> (25, -34)
  line L3 (25, -34) -> (25, 0)
  line L4 (25, 0) -> (0, 0)
  line L5 (0, 0) -> (0, -1.5369)
  line L6 (0, 9) -> (5, 9)
  line L7 (5, 9) -> (5, -1.5369)
  line L8 (5, -1.5369) -> (0, -1.5369)
  line L9 (0, -1.5369) -> (0, 9)
  constraint horizontal L6
  constraint vertical L7
  constraint horizontal L8
  constraint vertical L9
  constraint coincident L0 L7.end
extrude "Extrude13" cut sketch "Sketch12" against normal blind 23 contours L0 L4 L5 L7 L8 L9 | L4 L6 L7 L9
sketch "Sketch13" plane through (0, 25, 0) normal (0, 1, 0) x (-1, 0, 0)
  line L0 (0, 9) -> (-5, 9)
  arc A0 (-14, 0) -> (-5, 9) centre (-14, 9) ccw
  line L1 (-14, 0) -> (-14, -34)
  line L2 (-14, -34) -> (9, -34)
  line L3 (9, -34) -> (9, 0)
  arc A1 (0, 9) -> (9, 0) centre (9, 9) ccw
  circle A2 centre (-2.5, -31.5) radius 1
  circle A3 centre (-2.5, -2.5) radius 1
  line L4 (-9, -29) -> (-9, -5)
  line L5 (-9, -5) -> (4, -5)
  line L6 (4, -5) -> (4, -29)
  line L7 (4, -29) -> (-9, -29)
sketch "Sketch14" plane through (-9, 0, 0) normal (-1, 0, 0) x (0, -1, 0)
  line L0 (-5, -1.5369) -> (-5, 0)
  line L1 (-5, 0) -> (-25, 0)
  line L2 (-25, 0) -> (-25, -34)
  line L3 (-25, -34) -> (-15, -34)
  line L4 (-15, -34) -> (-15, -1.5369)
  line L5 (-15, -1.5369) -> (-5, -1.5369)
  line L6 (-20, 9) -> (-25, 9)
  line L7 (-25, 9) -> (-25, 4)
  line L8 (-25, 4) -> (-20, 4)
  line L9 (-20, 4) -> (-20, 9)
  dimension "d51" = 5
  constraint horizontal L6
  constraint vertical L7
  constraint horizontal L8
  constraint vertical L9
  measures "d51" distance of L6.start L8.end
extrude "Extrude14" cut sketch "Sketch14" against normal blind 16 contours L6 L7 L8 L9
fillet "Fillet3" radius 5.5 1 edges at (2.5, 25, 4)
sketch "Sketch15" plane through (-9, 0, 0) normal (-1, 0, 0) x (0, -1, 0)
  arc A0 (-24.7979, 0) -> (-25, -1.4772) centre (-19.5, -1.4772) ccw
  line L0 (-25, -1.4772) -> (-25, -34)
  line L1 (-25, -34) -> (-15, -34)
  line L2 (-15, -34) -> (-15, -1.5369)
  line L3 (-15, -1.5369) -> (-5, -1.5369)
  line L4 (-5, -1.5369) -> (-5, 0)
  line L5 (-5, 0) -> (-24.7979, 0)
  line L6 (-23, -3) -> (-17, -3)
  line L7 (-17, -3) -> (-17, -31)
  line L8 (-17, -31) -> (-23, -31)
  line L9 (-23, -31) -> (-23, -3)
  dimension "d62" = 2
  constraint horizontal L6
  constraint vertical L7
  constraint horizontal L8
  constraint vertical L9
  measures "d62" distance of L2 L7
extrude "Extrude15" add sketch "Sketch15" along normal blind 6 contours L6 L7 L8 L9
sketch "Sketch16" plane through (0, 17, 0) normal (0, -1, 0) x (1, 0, 0)
  line L0 (-9, -31) -> (-9, -3)
  line L1 (-9, -3) -> (-15, -3)
  line L2 (-15, -3) -> (-15, -31)
  line L3 (-15, -31) -> (-9, -31)
  line L4 (-9, -3) -> (-12, -3)
  line L5 (-12, -3) -> (-12, -31)
  line L6 (-12, -31) -> (-9, -31)
  line L7 (-9, -31) -> (-9, -3)
  constraint horizontal L4
  constraint vertical L5
  constraint horizontal L6
  constraint vertical L7
  constraint midpoint L3 L5.end
  constraint coincident L0.end L1.start
extrude "Extrude16" [suppressed]
sketch "Sketch17" plane through (0, 0, -3) normal (0, 0, 1) x (-1, 0, 0)
  line L0 (12, -21) -> (9, -21)
  line L1 (9, -21) -> (9, -23)
  line L2 (9, -23) -> (15, -23)
  line L3 (15, -23) -> (15, -17)
  line L4 (15, -17) -> (12, -17)
  line L5 (12, -17) -> (12, -21)
  line L6 (12, -21) -> (13.9977, -21)
  line L7 (13.9977, -21) -> (13.9977, -19)
  line L8 (13.9977, -19) -> (12, -19)
  line L9 (12, -19) -> (12, -21)
  constraint horizontal L6
  constraint vertical L7
  constraint horizontal L8
  constraint vertical L9
  constraint coincident L0.start L5.end
extrude "Extrude17" [suppressed]

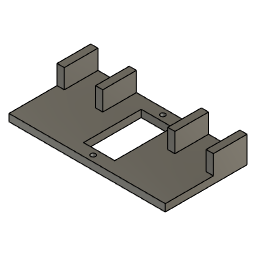
design "extras_plate"
Autodesk Fusion 360 part; units mm, degrees
sketch "Sketch1" plane through (0, 0, 0) normal (0, 0, 1) x (1, 0, 0)
  line L0 (0, 0) -> (65, 0)
  line L1 (65, 0) -> (65, 34)
  line L2 (65, 34) -> (0, 34)
  line L3 (0, 34) -> (0, 0)
  dimension "d1" = 65
  dimension "d2" = 34
  constraint horizontal L0
  constraint vertical L1
  constraint horizontal L2
  constraint vertical L3
  constraint coincident L0.start L3.end
  measures "d1" distance of L0.start L0.end
  measures "d2" distance of L0.start L2.end
extrude "Extrude1" add sketch "Sketch1" along normal blind 3
sketch "Sketch2" plane through (0, 0, 3) normal (0, 0, 1) x (-1, 0, 0)
  line L0 (0, -34) -> (0, 0)
  line L1 (0, 0) -> (-65, 0)
  line L2 (-65, 0) -> (-65, -34)
  line L3 (-65, -34) -> (0, -34)
  line L4 (0, -34) -> (-3, -34)
  line L5 (-3, -34) -> (-16, -34)
  line L6 (-16, -34) -> (-19, -34)
  line L7 (-65, -34) -> (-62, -34)
  line L8 (-62, -34) -> (-49, -34)
  line L9 (-49, -34) -> (-46, -34)
  line L10 (0, -34) -> (-3, -34)
  line L11 (-3, -34) -> (-3, -20)
  line L12 (-3, -20) -> (0, -20)
  line L13 (0, -20) -> (0, -34)
  line L14 (-16, -34) -> (-19, -34)
  line L15 (-19, -34) -> (-19, -20)
  line L16 (-19, -20) -> (-16, -20)
  line L17 (-16, -20) -> (-16, -34)
  line L18 (-49, -34) -> (-46, -34)
  line L19 (-46, -34) -> (-46, -20)
  line L20 (-46, -20) -> (-49, -20)
  line L21 (-49, -20) -> (-49, -34)
  line L22 (-62, -34) -> (-65, -34)
  line L23 (-65, -34) -> (-65, -20)
  line L24 (-65, -20) -> (-62, -20)
  line L25 (-62, -20) -> (-62, -34)
  dimension "d5" = 3
  dimension "d6" = 13
  dimension "d7" = 3
  dimension "d8" = 3
  dimension "d9" = 13
  dimension "d10" = 3
  dimension "d11" = 3
  dimension "d12" = 14
  dimension "d13" = 3
  dimension "d14" = 14
  dimension "d15" = 3
  dimension "d16" = 14
  dimension "d17" = 14
  constraint coincident L0.start L3.end
  constraint perpendicular L0 L4
  constraint parallel L3 L5
  constraint parallel L3 L6
  constraint coincident L2.end L3.start
  constraint perpendicular L2 L7
  constraint parallel L3 L8
  constraint parallel L3 L9
  constraint horizontal L10
  constraint vertical L11
  constraint horizontal L12
  constraint vertical L13
  constraint horizontal L14
  constraint vertical L15
  constraint horizontal L16
  constraint vertical L17
  constraint horizontal L18
  constraint vertical L19
  constraint horizontal L20
  constraint vertical L21
  constraint horizontal L22
  constraint vertical L23
  constraint horizontal L24
  constraint vertical L25
  measures "d5" distance of L0.start L4.end
  measures "d6" distance of L4.end L5.end
  measures "d7" distance of L5.end L6.end
  measures "d8" distance of L2.end L7.end
  measures "d9" distance of L7.end L8.end
  measures "d10" distance of L8.end L9.end
  measures "d11" distance of L0.start L4.end
  measures "d12" distance of L0.start L12.end
  measures "d13" distance of L5.end L6.end
  measures "d14" distance of L5.end L16.end
  measures "d15" distance of L8.end L9.end
  measures "d16" distance of L8.end L20.end
  measures "d17" distance of L7.end L24.end
extrude "Extrude2" add sketch "Sketch2" along normal blind 8 contours L0 L3 L4 L10 L11 L12 L13 | L3 L6 L14 L15 L16 L17 | L2 L3 L7 L22 L23 L24 L25 | L3 L9 L18 L19 L20 L21
sketch "Sketch3" plane through (0, 0, 3) normal (0, 0, 1) x (-1, 0, 0)
  line L0 (-3, -34) -> (-3, -20)
  line L1 (-3, -20) -> (0, -20)
  line L2 (0, -20) -> (0, 0)
  line L3 (0, 0) -> (-65, 0)
  line L4 (-65, 0) -> (-65, -20)
  line L5 (-65, -20) -> (-62, -20)
  line L6 (-62, -20) -> (-62, -34)
  line L7 (-62, -34) -> (-49, -34)
  line L8 (-49, -34) -> (-49, -20)
  line L9 (-49, -20) -> (-46, -20)
  line L10 (-46, -20) -> (-46, -34)
  line L11 (-46, -34) -> (-19, -34)
  line L12 (-19, -34) -> (-19, -20)
  line L13 (-19, -20) -> (-16, -20)
  line L14 (-16, -20) -> (-16, -34)
  line L15 (-16, -34) -> (-3, -34)
  line L16 (-32.5, -34) -> (-32.5, 0)
  line L17 (-32.5, -17) -> (-45, -17)
  line L18 (-32.5, -17) -> (-39, -17)
  line L19 (-39, -17) -> (-39, -29)
  line L20 (-39, -29) -> (-32.5, -29)
  line L21 (-32.5, -29) -> (-32.5, -17)
  line L22 (-39, -29) -> (-26, -29)
  line L23 (-26, -29) -> (-26, -5)
  line L24 (-26, -5) -> (-39, -5)
  line L25 (-39, -5) -> (-39, -29)
  line L26 (-32.5, -29) -> (-32.5, -31.5)
  line L27 (-32.5, -5) -> (-32.5, -2.5)
  circle A0 centre (-32.5, -31.5) radius 1
  circle A1 centre (-32.5, -2.5) radius 1
  dimension "d20" = 6.5
  dimension "d21" = 12
  dimension "d22" = 24
  dimension "d23" = 2.5
  dimension "d24" = 2.5
  dimension "d25" = 2
  dimension "d26" = 2
  constraint midpoint L11 L16.start
  constraint midpoint L3 L16.end
  constraint midpoint L16 L17.start
  constraint perpendicular L16 L17
  constraint horizontal L18
  constraint vertical L19
  constraint horizontal L20
  constraint vertical L21
  constraint horizontal L22
  constraint vertical L23
  constraint horizontal L24
  constraint vertical L25
  constraint coincident L20 L19.end
  constraint coincident L19 L20.start
  constraint perpendicular L22 L26
  constraint midpoint L24 L27.start
  constraint perpendicular L24 L27
  constraint coincident L26.end A0.centre
  constraint coincident L27.end A1.centre
  measures "d20" distance of L17.start L18.end
  measures "d21" distance of L17.start L20.end
  measures "d22" distance of L19.end L24.end
  measures "d23" distance of L20.end L26.end
  measures "d24" distance of L27.start L27.end
  measures "d25" diameter of A0
  measures "d26" diameter of A1
extrude "Extrude3" cut sketch "Sketch3" against normal blind 3 contours L16 L27 A1 | L16 L27 A1 | L16 L26 A0 | L16 L26 A0 | L16 L21 L22 L23 L24 | L16 L17 L18 L24 L25 | L16 L17 L18 L19 L20 L21 L22 L25

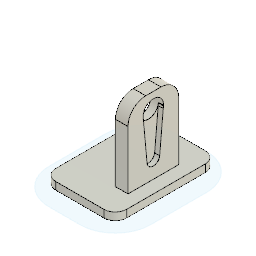
design "smaller_foot"
Autodesk Fusion 360 part; units mm, degrees
sketch "Sketch1" plane through (0, 0, 0) normal (0, 0, 1) x (1, 0, 0)
  line L0 (0, 0) -> (40, 0)
  line L1 (40, 0) -> (40, 50)
  line L2 (40, 50) -> (0, 50)
  line L3 (0, 50) -> (0, 0)
  constraint horizontal L0
  constraint vertical L1
  constraint horizontal L2
  constraint vertical L3
  constraint coincident L0.start L3.end
extrude "Extrude1" add sketch "Sketch1" along normal blind 5
sketch "Sketch6" plane through (0, 0, 5) normal (0, 0, 1) x (-1, 0, 0)
  line L0 (0, -50) -> (0, 0)
  line L1 (0, 0) -> (-40, 0)
  line L2 (-40, 0) -> (-40, -50)
  line L3 (-40, -50) -> (0, -50)
  line L4 (-30, -40) -> (-25, -40)
  line L5 (-25, -40) -> (-25, -10)
  line L6 (-25, -10) -> (-30, -10)
  line L7 (-30, -10) -> (-30, -40)
  constraint horizontal L4
  constraint vertical L5
  constraint horizontal L6
  constraint vertical L7
extrude "Extrude4" add sketch "Sketch6" along normal blind 32 contours L4 L5 L6 L7
sketch "Sketch7" plane through (30, 0, 0) normal (1, 0, 0) x (0, 1, 0)
  line L0 (10, 5) -> (40, 5)
  line L1 (40, 5) -> (40, 37)
  line L2 (40, 37) -> (10, 37)
  line L3 (10, 37) -> (10, 5)
  circle A0 centre (25, 12) radius 2
  circle A1 centre (25, 28) radius 4
  line L4 (28.9999, 28.0281) -> (26.9848, 11.7542)
  line L5 (23.0152, 11.7542) -> (21.0001, 28.0281)
  dimension "d22" = 4
  dimension "d23" = 8
  constraint coincident A1 L4.start
  constraint coincident A0 L4.end
  constraint tangent A0 L4
  constraint coincident A0 L5.start
  constraint coincident A1 L5.end
  constraint tangent A0 L5
  measures "d22" diameter of A0
  measures "d23" diameter of A1
extrude "Extrude5" cut sketch "Sketch7" against normal blind 2 contours A0 | A0 A1 L4 L5 | A1 L4 L5
fillet "Fillet1" radius 6 2 edges at (27.5, 10, 37) (27.5, 40, 37)
fillet "Fillet2" radius 14 4 edges at (40, 0, 2.5) (40, 50, 2.5) (0, 50, 2.5) (0, 0, 2.5)
sketch "Sketch8" plane through (28, 0, 0) normal (1, 0, 0) x (0, 1, 0)
  arc A0 (28.9999, 28.0281) -> (21.0001, 28.0281) centre (25, 28) ccw
  line L0 (21.0001, 28.0281) -> (23.0152, 11.7542)
  arc A1 (23.0152, 11.7542) -> (26.9848, 11.7542) centre (25, 12) ccw
  line L1 (26.9848, 11.7542) -> (28.9999, 28.0281)
  circle A2 centre (25, 28) radius 4
  constraint concentric A0 A2
extrude "Extrude6" cut sketch "Sketch8" against normal blind 3 contours A0 L0 L1 A2
sketch "Sketch9" plane through (30, 0, 0) normal (1, 0, 0) x (0, 1, 0)
  arc A0 (40, 31) -> (34, 37) centre (34, 31) ccw
  line L0 (34, 37) -> (16, 37)
  arc A1 (16, 37) -> (10, 31) centre (16, 31) ccw
  line L1 (10, 31) -> (10, 5)
  line L2 (10, 5) -> (40, 5)
  line L3 (40, 5) -> (40, 31)
  line L4 (23.0152, 11.7542) -> (21.0001, 28.0281)
  arc A2 (28.9999, 28.0281) -> (21.0001, 28.0281) centre (25, 28) ccw
  line L5 (28.9999, 28.0281) -> (26.9848, 11.7542)
  arc A3 (23.0152, 11.7542) -> (26.9848, 11.7542) centre (25, 12) ccw
  circle A4 centre (25, 12) radius 2.5
  line L6 (25, 9.5) -> (25, 32.5)
  line L7 (25, 32.5) -> (25, 28.5)
  circle A5 centre (25, 28.5) radius 4
  line L8 (21.0001, 28.0281) -> (22.5107, 11.7687)
  line L9 (27.4893, 11.7687) -> (28.9922, 28.25)
  dimension "d32" = 5
  dimension "d33" = 23
  dimension "d34" = 4
  dimension "d35" = 8
  constraint concentric A3 A4
  constraint coincident A4 L6.start
  constraint vertical L6
  constraint parallel L6 L7
  constraint coincident L7.end A5.centre
  constraint coincident L4.end A2.end
  constraint coincident A4 L8.end
  constraint tangent A4 L8
  constraint coincident A4 L9.start
  constraint coincident A2 L9.end
  constraint coincident A5 L9.end
  measures "d32" diameter of A4
  measures "d33" distance of L6.start L6.end
  measures "d34" distance of L6.end L7.end
  measures "d35" diameter of A5
extrude "Extrude7" cut sketch "Sketch9" against normal blind 5 contours L4 A3 A4 L6 | L4 A3 A4 L6 | L4 A4 L8 | L4 A2 A4 L6 A5 | L5 A3 A4 L6 | L5 A4 L9 | L5 A3 A4 L6 | L5 A4 L6 A5 L9 | A2 L6 L7 A5 | A2 L6 L7 A5 picked at (24.2303, 32.2478) picked at (25.7476, 32.2532)